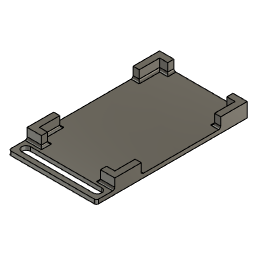
DC-DC Converter Case (Autodesk Fusion 360 design; units mm, degrees)
Autodesk Fusion 360 part; units mm, degrees
sketch "Sketch1" plane through (0, 0, 0) normal (0, 0, 1) x (1, 0, 0)
  line L0 (18.5, 29.5) -> (-18.5, 29.5) construction
  line L1 (-18.5, 29.5) -> (-18.5, -29.5) construction
  line L2 (-18.5, -29.5) -> (18.5, -29.5) construction
  line L3 (18.5, -29.5) -> (18.5, 29.5) construction
  line L4 (18.5, 29.5) -> (-18.5, -29.5) construction
  line L5 (-18.5, 29.5) -> (18.5, -29.5) construction
  line L6 (-18.5, 19.5) -> (-21.5, 19.5)
  line L7 (-21.5, 19.5) -> (-21.5, 32.5)
  line L8 (-21.5, 32.5) -> (-14.5, 32.5)
  line L9 (-14.5, 32.5) -> (-14.5, 29.5)
  line L10 (0, 29.5) -> (0, -29.5) construction
  line L11 (21.5, 32.5) -> (14.5, 32.5)
  line L12 (21.5, 19.5) -> (21.5, 32.5)
  line L13 (18.5, 19.5) -> (21.5, 19.5)
  line L14 (14.5, 32.5) -> (14.5, 29.5)
  line L15 (-18.5, 0) -> (18.5, 0) construction
  line L16 (-18.5, -19.5) -> (-21.5, -19.5)
  line L17 (-21.5, -19.5) -> (-21.5, -32.5)
  line L18 (-21.5, -32.5) -> (-14.5, -32.5)
  line L19 (-14.5, -32.5) -> (-14.5, -29.5)
  line L20 (21.5, -32.5) -> (14.5, -32.5)
  line L21 (14.5, -32.5) -> (14.5, -29.5)
  line L22 (21.5, -19.5) -> (21.5, -32.5)
  line L23 (18.5, -19.5) -> (21.5, -19.5)
  line L24 (14.5, 29.5) -> (18.5, 29.5)
  line L25 (18.5, 19.5) -> (18.5, 29.5)
  line L26 (-18.5, 29.5) -> (-18.5, 19.5)
  line L27 (-18.5, 29.5) -> (-14.5, 29.5)
  line L28 (-18.5, -19.5) -> (-18.5, -29.5)
  line L29 (-14.5, -29.5) -> (-18.5, -29.5)
  line L30 (14.5, -29.5) -> (18.5, -29.5)
  line L31 (18.5, -29.5) -> (18.5, -19.5)
  dimension "d1" = 59
  dimension "d2" = 37
  dimension "d3" = 13
  dimension "d4" = 3
  dimension "d5" = 4
  dimension "d6" = 3
  constraint horizontal L0
  constraint perpendicular L0 L1
  constraint parallel L0 L2
  constraint parallel L1 L3
  constraint coincident L4 origin
  constraint coincident L5 origin
  constraint coincident L1 L6.start
  constraint perpendicular L1 L6
  constraint perpendicular L6 L7
  constraint perpendicular L7 L8
  constraint coincident L0 L9.end
  constraint perpendicular L0 L9
  constraint midpoint L0 L10.start
  constraint midpoint L2 L10.end
  constraint symmetric L6.start L10 L13.start
  constraint symmetric L6.end L10 L12.start
  constraint symmetric L7.end L10 L11.start
  constraint symmetric L8.end L10 L11.end
  constraint symmetric L9.end L10 L14.end
  constraint midpoint L1 L15.start
  constraint midpoint L3 L15.end
  constraint symmetric L6.start L15 L16.start
  constraint symmetric L6.end L15 L16.end
  constraint symmetric L7.end L15 L17.end
  constraint symmetric L8.end L15 L18.end
  constraint symmetric L9.end L15 L19.end
  constraint symmetric L11.start L15 L20.start
  constraint symmetric L11.end L15 L20.end
  constraint symmetric L12.start L15 L22.start
  constraint symmetric L13.start L15 L23.start
  constraint symmetric L14.end L15 L21.end
  measures "d1" distance of L0.start L2.end
  measures "d2" distance of L1.end L2.end
  measures "d3" distance of L6.end L7.end
  measures "d4" distance of L6.start L6.end
  measures "d5" distance of L1 L9
  measures "d6" distance of L8.end L9.end
extrude "Extrude1" add sketch "Sketch1" along normal blind 5 makes body 1 at (-21.5, 23.8333, 1.6667) makes body 2 at (-21.5, -23.8333, 1.6667) makes body 3 at (21.5, 23.8333, 1.6667) makes body 4 at (21.5, -23.8333, 1.6667)
sketch "Sketch2" plane through (0, 0, 0) normal (0, 0, -1) x (1, 0, 0)
  line L0 (-21.5, 19.5) -> (-18.5, 19.5)
  line L1 (-18.5, 19.5) -> (-18.5, 29.5)
  line L2 (-18.5, 29.5) -> (-14.5, 29.5)
  line L3 (-14.5, 29.5) -> (-14.5, 32.5)
  line L4 (-14.5, 32.5) -> (-21.5, 32.5)
  line L5 (-21.5, 32.5) -> (-21.5, 19.5)
  line L6 (-21.5, 32.5) -> (21.5, 32.5) construction
  line L7 (21.5, 32.5) -> (21.5, -32.5)
  line L8 (21.5, -32.5) -> (-21.5, -32.5)
  line L9 (-21.5, -32.5) -> (-21.5, 32.5)
  line L10 (5, 32.5) -> (-5, 32.5) construction
  line L11 (0, -32.5) -> (0, 32.5) construction
  line L12 (21.5, 32.5) -> (-21.5, 32.5)
  line L13 (-21.5, 32.5) -> (-21.5, 41.5)
  line L14 (-21.5, 41.5) -> (21.5, 41.5)
  line L15 (21.5, 41.5) -> (21.5, 32.5)
  line L16 (21.5, 37) -> (-21.5, 37) construction
  line L17 (0, 32.5) -> (0, 41.5) construction
  line L18 (17.5, 39.15) -> (-17.5, 39.15)
  arc A0 (-17.5, 39.15) -> (-17.5, 34.85) centre (-17.5, 37) ccw
  line L19 (-17.5, 34.85) -> (17.5, 34.85)
  arc A1 (17.5, 34.85) -> (17.5, 39.15) centre (17.5, 37) ccw
  line L20 (17.5, 37) -> (-17.5, 37) construction
  point P0 (0, 37)
  dimension "d9" = 10
  dimension "d10" = 9
  dimension "d11" = 35
  dimension "d12" = 4.3
  constraint horizontal L6
  constraint vertical L7
  constraint horizontal L8
  constraint vertical L9
  constraint coincident L4.end L5.start
  constraint horizontal L10
  constraint midpoint L8 L11.start
  constraint midpoint L6 L11.end
  constraint midpoint L10 L11.end
  constraint horizontal L12
  constraint vertical L13
  constraint horizontal L14
  constraint vertical L15
  constraint midpoint L15 L16.start
  constraint midpoint L13 L16.end
  constraint midpoint origin L11
  constraint collinear L9 L13
  constraint midpoint L14 L17.end
  constraint tangent L18 A0
  constraint tangent A0 L19
  constraint parallel L18 L19
  constraint tangent L19 A1
  constraint tangent L18 A1
  constraint coincident L16 A0.centre
  constraint perpendicular L17 L20
  constraint midpoint L16 P0
  constraint midpoint L20 P0
  measures "d9" distance of L10.start L10.end
  measures "d10" distance of L4.end L13.end
  measures "d11" distance of A1.centre A0.centre
  measures "d12" distance of L18 L19
extrude "Extrude2" add sketch "Sketch2" along normal blind 2 bodies 1 2 3 4
fillet "Fillet1" radius 1 16 edges at (-20, 19.5, 0) (-18.5, 24.5, 0) (-16.5, 29.5, 0) (-14.5, 31, 0) (14.5, 31, 0) (16.5, 29.5, 0) (18.5, 24.5, 0) (20, 19.5, 0) (20, -19.5, 0) (18.5, -24.5, 0) (16.5, -29.5, 0) (14.5, -31, 0) (-14.5, -31, 0) (-16.5, -29.5, 0) (-18.5, -24.5, 0) (-20, -19.5, 0) on bodies 1
fillet "Fillet1" radius 1 4 edges at (-21.5, -41.5, -1) (21.5, -41.5, -1) (18, -32.5, 0) (-18, -32.5, 0) on bodies 1
